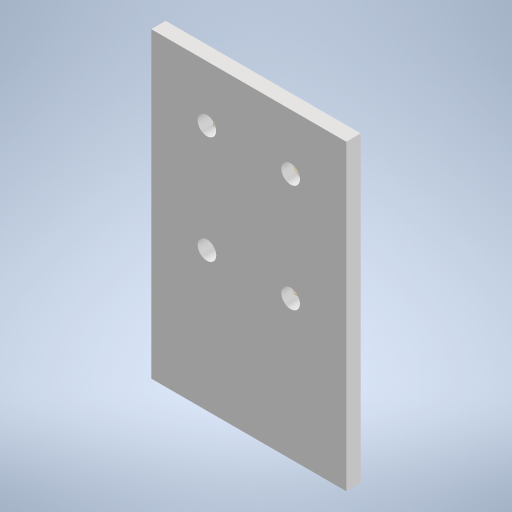
# Autodesk Inventor part: _Tooling_PCBPaste
Saved by Autodesk Inventor 2023.2 (Build 272271030, 271C)
## iProperties
Created: 2023-03-08
Part Number: _Tooling_PCBPaste
Material: Generic
Document SubType Name: Modeling
Designer: atrus
Density: 1 g/cm^3
Appearance: Default
Author: atrus
Autodesk Inventor part; units mm, degrees
ref_plane "YZ Plane" through (0, 0, 0) normal (1, 0, 0) x (0, 1, 0)
ref_plane "XZ Plane" through (0, 0, 0) normal (0, 1, 0) x (-1, 0, 0)
ref_plane "XY Plane" through (0, 0, 0) normal (0, 0, 1) x (1, 0, 0)
ref_plane "Work Plane1" through (0, 0, 0) normal (0, 0, 1) x (1, 0, 0)
sketch "Sketch1" plane through (0, 0, 0) normal (0, 0, 1) x (1, 0, 0)
  circle A0 centre (15.9836, 21.7327) radius 1.632 construction
  circle A1 centre (-16.0164, 21.7327) radius 1.632 construction
  circle A2 centre (15.9836, -10.6173) radius 1.632 construction
  circle A3 centre (-16.0164, -10.6173) radius 1.632 construction
  line L0 (19, -24.5) -> (19, 24.5) construction
  line L1 (19, 24.5) -> (-19, 24.5) construction
  line L2 (-19, 24.5) -> (-19, -24.5) construction
  line L3 (-19, -24.5) -> (19, -24.5) construction
  line L4 (-19.1, 24.6) -> (19.1, 24.6)
  line L5 (19.1, 24.6) -> (19.1, -24.6)
  line L6 (19.1, -24.6) -> (-19.1, -24.6)
  line L7 (-19.1, -24.6) -> (-19.1, 24.6)
  circle A4 centre (-16.0164, 21.7327) radius 1.5319
  circle A5 centre (15.9836, 21.7327) radius 1.5319
  circle A6 centre (-16.0164, -10.6173) radius 1.5319
  circle A7 centre (15.9836, -10.6173) radius 1.5319
  line L8 (-44.5, 50) -> (44.5, 50)
  line L9 (44.5, 50) -> (44.5, -88.1)
  line L10 (44.5, -88.1) -> (-44.5, -88.1)
  line L11 (-44.5, -88.1) -> (-44.5, 50)
  point P0 (0, 0)
  dimension "d0" = 0.1
  dimension "d1" = 0.1
  dimension "d2" = 0.1
  dimension "d3" = 0.1
  dimension "d4" = 0.1
  dimension "d5" = 63.5
  dimension "d6" = 25.4
  dimension "d7" = 25.4
  dimension "d8" = 25.4
  constraints: 16 end point, 4 centre point, 2 parallel, 1 horizontal, 1 perpendicular, 3 other
  measures "d0" distance between parallel lines of L1 L4
  measures "d1" radial gap between concentric circles of A1 A4
  measures "d2" radial gap between concentric circles of A0 A5
  measures "d3" radial gap between concentric circles of A3 A6
  measures "d4" radial gap between concentric circles of A2 A7
  measures "d5" distance between parallel lines of L10 L6
  measures "d6" distance between parallel lines of L8 L4
  measures "d7" distance between parallel lines of L9 L5
  measures "d8" distance between parallel lines of L11 L7
extrude "Extrusion1" add sketch "Sketch1" against normal blind 1.6
sketch "Sketch2" plane through (0, 0, 0) normal (0, 0, 1) x (1, 0, 0)
  line L0 (-44.5, 50) -> (44.5, 50) projected
  line L1 (44.5, 50) -> (44.5, -88.1) projected
  line L2 (-44.5, 50) -> (44.5, 50)
  line L3 (44.5, 50) -> (44.5, -88.1)
  line L4 (44.5, -88.1) -> (-44.5, -88.1)
  line L5 (-44.5, -88.1) -> (-44.5, 50)
  point P0 (0, 0)
  constraints: 8 end point, 2 parallel, 1 horizontal, 1 perpendicular
extrude "Extrusion2" add sketch "Sketch2" along normal blind 5
sketch "Sketch3" plane through (0, 0, -1.6) normal (0, 0, -1) x (-1, 0, 0)
  line L0 (-19.1, 24.6) -> (-19.1, -24.6) projected
  circle A0 centre (-15.9836, 21.7327) radius 1.5319 projected
  circle A1 centre (-19.1, 24.6) radius 4.2348
  line L1 (-19.1, 24.6) -> (19.1, 24.6) projected
  circle A2 centre (16.0164, 21.7327) radius 1.5319 projected
  circle A3 centre (19.1, 24.6) radius 4.2107
  circle A4 centre (19.1, -24.6) radius 4.2348
  circle A5 centre (-19.1, -24.6) radius 4.2348
  point P0 (0, 0)
  constraints: 2 centre point, 1 coincident, 8 other
extrude "Extrusion3" cut sketch "Sketch3" against normal through all contours L1 A1 A0 L0 | L0 A1 L1 | A0 A1 | A2 A3 | A2 A3 | A4 | A5 picked at (-16.3746, 22.0925) picked at (16.4181, 22.0806) picked at (20.3065, 26.0638)
sketch "Sketch4" plane through (0, 0, -1.6) normal (0, 0, -1) x (-1, 0, 0)
  line L0 (37.9315, -14.1978) -> (37.9315, 20.0606) construction
  line L1 (37.9315, 20.0606) -> (45.2777, 20.0606) construction
  line L2 (45.2777, 20.0606) -> (45.2777, -14.1978) construction
  line L3 (45.2777, -14.1978) -> (37.9315, -14.1978) construction
  line L4 (41.1606, -12.3998) -> (39.2658, -13.2505)
  line L5 (39.2658, -13.2505) -> (38.859, -13.4268)
  line L6 (38.859, -13.4268) -> (40.1734, -13.4268)
  line L7 (40.1734, -13.4268) -> (41.1606, -13.4268)
  line L8 (41.1606, -13.4268) -> (41.1606, -13.9702)
  line L9 (41.1606, -13.9702) -> (37.9856, -13.9702)
  line L10 (37.9856, -13.9702) -> (37.9856, -13.2362)
  line L11 (37.9856, -13.2362) -> (39.8917, -12.3685)
  line L12 (39.8917, -12.3685) -> (40.2644, -12.2149)
  line L13 (40.2644, -12.2149) -> (38.8618, -12.2149)
  line L14 (38.8618, -12.2149) -> (37.9856, -12.2149)
  line L15 (37.9856, -12.2149) -> (37.9856, -11.6715)
  line L16 (37.9856, -11.6715) -> (41.1606, -11.6715)
  line L17 (41.1606, -11.6715) -> (41.1606, -12.3998)
  line L18 (41.1606, -9.5747) -> (40.8391, -9.589)
  spline S0 degree 2 poles (40.8391, -9.589) (40.9216, -9.6686) (41.0582, -9.8365) (41.1606, -10.0413) (41.2175, -10.2831) (41.2175, -10.4254) knots 0 0 0 1 2 3 4 4 4
  spline S1 degree 2 poles (41.2175, -10.4254) (41.2175, -10.616) (41.1065, -10.9033) (40.9074, -11.0968) (40.6229, -11.1964) (40.455, -11.1964) knots 0 0 0 1 2 3 4 4 4
  spline S2 degree 2 poles (40.455, -11.1964) (40.2786, -11.1964) (39.9827, -11.0484) (39.7694, -10.744) (39.647, -10.2888) (39.647, -9.9844) knots 0 0 0 1 2 3 4 4 4
  line L19 (39.647, -9.9844) -> (39.647, -9.6601)
  line L20 (39.647, -9.6601) -> (39.4991, -9.6601)
  spline S3 degree 2 poles (39.4991, -9.6601) (39.4052, -9.6601) (39.2516, -9.7141) (39.1435, -9.8336) (39.0866, -10.0214) (39.0866, -10.1608) knots 0 0 0 1 2 3 4 4 4
  spline S4 degree 2 poles (39.0866, -10.1608) (39.0866, -10.3799) (39.1862, -10.8038) (39.2772, -11.0029) knots 0 0 0 1 2 2 2
  line L21 (39.2772, -11.0029) -> (38.8021, -11.0029)
  spline S5 degree 2 poles (38.8021, -11.0029) (38.731, -10.8265) (38.6399, -10.3628) (38.6399, -10.1124) knots 0 0 0 1 2 2 2
  spline S6 degree 2 poles (38.6399, -10.1124) (38.6399, -9.8365) (38.7452, -9.4439) (38.9529, -9.1907) (39.2658, -9.0683) (39.4763, -9.0683) knots 0 0 0 1 2 3 4 4 4
  line L22 (39.4763, -9.0683) -> (41.1606, -9.0683)
  line L23 (41.1606, -9.0683) -> (41.1606, -9.5747)
  line L24 (40.0709, -9.6601) -> (40.0709, -10.0214)
  spline S7 degree 2 poles (40.0709, -10.0214) (40.0709, -10.1722) (40.1278, -10.3827) (40.2303, -10.5136) (40.364, -10.5733) (40.4408, -10.5733) knots 0 0 0 1 2 3 4 4 4
  spline S8 degree 2 poles (40.4408, -10.5733) (40.5916, -10.5733) (40.748, -10.3799) (40.748, -10.212) knots 0 0 0 1 2 2 2
  spline S9 degree 2 poles (40.748, -10.212) (40.748, -10.0868) (40.5688, -9.8194) (40.401, -9.6601) knots 0 0 0 1 2 2 2
  line L25 (40.401, -9.6601) -> (40.0709, -9.6601)
  line L26 (41.1606, -6.9118) -> (39.5532, -6.9118)
  spline S10 degree 2 poles (39.5532, -6.9118) (39.1463, -6.9118) (39.1463, -7.2134) knots 0 0 0 1 1 1
  spline S11 degree 2 poles (39.1463, -7.2134) (39.1463, -7.3642) (39.3881, -7.6401) (39.5987, -7.7938) knots 0 0 0 1 2 2 2
  line L27 (39.5987, -7.7938) -> (41.1606, -7.7938)
  line L28 (41.1606, -7.7938) -> (41.1606, -8.3855)
  line L29 (41.1606, -8.3855) -> (38.6911, -8.3855)
  line L30 (38.6911, -8.3855) -> (38.6911, -7.8734)
  line L31 (38.6911, -7.8734) -> (39.0553, -7.8592)
  spline S12 degree 2 poles (39.0553, -7.8592) (38.9614, -7.7852) (38.8078, -7.6202) (38.6968, -7.4325) (38.6399, -7.2134) (38.6399, -7.0768) knots 0 0 0 1 2 3 4 4 4
  spline S13 degree 2 poles (38.6399, -7.0768) (38.6399, -6.8862) (38.7651, -6.6046) (38.9898, -6.414) (39.3085, -6.3201) (39.5048, -6.3201) knots 0 0 0 1 2 3 4 4 4
  line L32 (39.5048, -6.3201) -> (41.1606, -6.3201)
  line L33 (41.1606, -6.3201) -> (41.1606, -6.9118)
  spline S14 degree 2 poles (39.9088, -3.4267) (40.199, -3.4267) (40.6826, -3.5917) (41.0269, -3.9018) (41.2175, -4.3542) (41.2175, -4.6444) knots 0 0 0 1 2 3 4 4 4
  spline S15 degree 2 poles (41.2175, -4.6444) (41.2175, -4.9203) (41.0582, -5.3528) (40.7395, -5.6543) (40.2616, -5.8137) (39.9429, -5.8137) knots 0 0 0 1 2 3 4 4 4
  spline S16 degree 2 poles (39.9429, -5.8137) (39.647, -5.8137) (39.1662, -5.6458) (38.8277, -5.3329) (38.6399, -4.8805) (38.6399, -4.596) knots 0 0 0 1 2 3 4 4 4
  spline S17 degree 2 poles (38.6399, -4.596) (38.6399, -4.3201) (38.8021, -3.8848) (39.1236, -3.586) (39.5958, -3.4267) (39.9088, -3.4267) knots 0 0 0 1 2 3 4 4 4
  spline S18 degree 2 poles (39.923, -4.0441) (39.5389, -4.0441) (39.152, -4.3343) (39.152, -4.6159) knots 0 0 0 1 2 2 2
  spline S19 degree 2 poles (39.152, -4.6159) (39.152, -4.7696) (39.2743, -4.9886) (39.4849, -5.1309) (39.7665, -5.1963) (39.9287, -5.1963) knots 0 0 0 1 2 3 4 4 4
  spline S20 degree 2 poles (39.9287, -5.1963) (40.3128, -5.1963) (40.7054, -4.8862) (40.7054, -4.6159) knots 0 0 0 1 2 2 2
  spline S21 degree 2 poles (40.7054, -4.6159) (40.7054, -4.468) (40.5859, -4.2489) (40.3754, -4.1124) (40.088, -4.0441) (39.923, -4.0441) knots 0 0 0 1 2 3 4 4 4
  line L34 (41.1606, -2.9374) -> (37.9856, -2.9374)
  line L35 (37.9856, -2.9374) -> (37.9856, -1.9132)
  spline S22 degree 2 poles (37.9856, -1.9132) (37.9856, -1.3698) (38.364, -0.8293) (38.748, -0.8293) knots 0 0 0 1 2 2 2
  spline S23 degree 2 poles (38.748, -0.8293) (38.8647, -0.8293) (39.0923, -0.8862) (39.28, -1.0028) (39.4251, -1.1763) (39.4678, -1.2958) knots 0 0 0 1 2 3 4 4 4
  spline S24 degree 2 poles (39.4678, -1.2958) (39.4877, -1.1763) (39.6015, -0.9601) (39.7836, -0.798) (40.0311, -0.7041) (40.1847, -0.7041) knots 0 0 0 1 2 3 4 4 4
  spline S25 degree 2 poles (40.1847, -0.7041) (40.6712, -0.7041) (41.1606, -1.3556) (41.1606, -1.9701) knots 0 0 0 1 2 2 2
  line L36 (41.1606, -1.9701) -> (41.1606, -2.9374)
  spline S26 degree 2 poles (40.6712, -1.9274) (40.6712, -1.7852) (40.5973, -1.569) (40.4692, -1.421) (40.2957, -1.347) (40.1961, -1.347) knots 0 0 0 1 2 3 4 4 4
  spline S27 degree 2 poles (40.1961, -1.347) (39.9884, -1.347) (39.7551, -1.6543) (39.7551, -1.9729) knots 0 0 0 1 2 2 2
  line L37 (39.7551, -1.9729) -> (39.7551, -2.3456)
  line L38 (39.7551, -2.3456) -> (40.6712, -2.3456)
  line L39 (40.6712, -2.3456) -> (40.6712, -1.9274)
  spline S28 degree 2 poles (38.8533, -1.4523) (38.7622, -1.4523) (38.6172, -1.5092) (38.5176, -1.6401) (38.4607, -1.8421) (38.4607, -1.9843) knots 0 0 0 1 2 3 4 4 4
  line L40 (38.4607, -1.9843) -> (38.4607, -2.3456)
  line L41 (38.4607, -2.3456) -> (39.2971, -2.3456)
  line L42 (39.2971, -2.3456) -> (39.2971, -1.9843)
  spline S29 degree 2 poles (39.2971, -1.9843) (39.2971, -1.8392) (39.226, -1.6372) (39.1036, -1.5092) (38.9443, -1.4523) (38.8533, -1.4523) knots 0 0 0 1 2 3 4 4 4
  spline S30 degree 2 poles (39.9088, 2.047) (40.199, 2.047) (40.6826, 1.882) (41.0269, 1.5719) (41.2175, 1.1196) (41.2175, 0.8294) knots 0 0 0 1 2 3 4 4 4
  spline S31 degree 2 poles (41.2175, 0.8294) (41.2175, 0.5534) (41.0582, 0.121) (40.7395, -0.1806) (40.2616, -0.3399) (39.9429, -0.3399) knots 0 0 0 1 2 3 4 4 4
  spline S32 degree 2 poles (39.9429, -0.3399) (39.647, -0.3399) (39.1662, -0.1721) (38.8277, 0.1409) (38.6399, 0.5932) (38.6399, 0.8777) knots 0 0 0 1 2 3 4 4 4
  spline S33 degree 2 poles (38.6399, 0.8777) (38.6399, 1.1537) (38.8021, 1.589) (39.1236, 1.8877) (39.5958, 2.047) (39.9088, 2.047) knots 0 0 0 1 2 3 4 4 4
  spline S34 degree 2 poles (39.923, 1.4297) (39.5389, 1.4297) (39.152, 1.1395) (39.152, 0.8578) knots 0 0 0 1 2 2 2
  spline S35 degree 2 poles (39.152, 0.8578) (39.152, 0.7042) (39.2743, 0.4851) (39.4849, 0.3429) (39.7665, 0.2774) (39.9287, 0.2774) knots 0 0 0 1 2 3 4 4 4
  spline S36 degree 2 poles (39.9287, 0.2774) (40.3128, 0.2774) (40.7054, 0.5875) (40.7054, 0.8578) knots 0 0 0 1 2 2 2
  spline S37 degree 2 poles (40.7054, 0.8578) (40.7054, 1.0058) (40.5859, 1.2248) (40.3754, 1.3614) (40.088, 1.4297) (39.923, 1.4297) knots 0 0 0 1 2 3 4 4 4
  line L43 (41.1606, 4.1495) -> (40.327, 3.589)
  line L44 (40.327, 3.589) -> (41.1606, 3.02)
  line L45 (41.1606, 3.02) -> (41.1606, 2.3059)
  line L46 (41.1606, 2.3059) -> (39.9173, 3.2277)
  line L47 (39.9173, 3.2277) -> (38.6911, 2.3543)
  line L48 (38.6911, 2.3543) -> (38.6911, 3.0769)
  line L49 (38.6911, 3.0769) -> (39.5048, 3.6288)
  line L50 (39.5048, 3.6288) -> (38.6911, 4.1751)
  line L51 (38.6911, 4.1751) -> (38.6911, 4.8408)
  line L52 (38.6911, 4.8408) -> (39.9116, 3.9901)
  line L53 (39.9116, 3.9901) -> (41.1606, 4.8863)
  line L54 (41.1606, 4.8863) -> (41.1606, 4.1495)
  line L55 (41.1606, 9.4155) -> (41.1606, 8.7327)
  line L56 (41.1606, 8.7327) -> (38.6911, 7.7569)
  line L57 (38.6911, 7.7569) -> (38.6911, 8.4169)
  line L58 (38.6911, 8.4169) -> (40.0937, 8.929)
  line L59 (40.0937, 8.929) -> (40.5461, 9.0827)
  line L60 (40.5461, 9.0827) -> (40.1108, 9.2334)
  line L61 (40.1108, 9.2334) -> (38.6911, 9.7512)
  line L62 (38.6911, 9.7512) -> (38.6911, 10.3885)
  line L63 (38.6911, 10.3885) -> (41.1606, 9.4155)
  spline S38 degree 2 poles (40.1904, 12.912) (40.4266, 12.912) (40.8021, 12.7385) (41.0667, 12.3743) (41.2089, 11.8252) (41.2089, 11.4554) knots 0 0 0 1 2 3 4 4 4
  spline S39 degree 2 poles (41.2089, 11.4554) (41.2089, 11.3729) (41.2004, 11.1908) (41.189, 11.0116) (41.1719, 10.8409) (41.1606, 10.7726) knots 0 0 0 1 2 3 4 4 4
  line L64 (41.1606, 10.7726) -> (40.6456, 10.7726)
  spline S40 degree 2 poles (40.6456, 10.7726) (40.6741, 10.9262) (40.7111, 11.3074) (40.7111, 11.5123) knots 0 0 0 1 2 2 2
  spline S41 degree 2 poles (40.7111, 11.5123) (40.7111, 11.7143) (40.6428, 12.0073) (40.5148, 12.1951) (40.3241, 12.2861) (40.2047, 12.2861) knots 0 0 0 1 2 3 4 4 4
  spline S42 degree 2 poles (40.2047, 12.2861) (40.1022, 12.2861) (39.9315, 12.1951) (39.812, 12.0045) (39.7466, 11.7114) (39.7466, 11.5094) knots 0 0 0 1 2 3 4 4 4
  line L65 (39.7466, 11.5094) -> (39.7466, 11.1567)
  line L66 (39.7466, 11.1567) -> (39.2943, 11.1567)
  line L67 (39.2943, 11.1567) -> (39.2943, 11.4781)
  spline S43 degree 2 poles (39.2943, 11.4781) (39.2943, 11.6687) (39.2203, 11.9191) (39.0923, 12.067) (38.9187, 12.1296) (38.8248, 12.1296) knots 0 0 0 1 2 3 4 4 4
  spline S44 degree 2 poles (38.8248, 12.1296) (38.6314, 12.1296) (38.4294, 11.8764) (38.4294, 11.6118) knots 0 0 0 1 2 2 2
  spline S45 degree 2 poles (38.4294, 11.6118) (38.4294, 11.4241) (38.5034, 11.0542) (38.5631, 10.8579) knots 0 0 0 1 2 2 2
  line L68 (38.5631, 10.8579) -> (38.0652, 10.8579)
  spline S46 degree 2 poles (38.0652, 10.8579) (38.0282, 10.966) (37.9799, 11.1652) (37.9457, 11.3643) (37.9315, 11.5692) (37.9315, 11.6773) knots 0 0 0 1 2 3 4 4 4
  spline S47 degree 2 poles (37.9315, 11.6773) (37.9315, 11.939) (38.0425, 12.3373) (38.2502, 12.6047) (38.546, 12.7413) (38.7281, 12.7413) knots 0 0 0 1 2 3 4 4 4
  spline S48 degree 2 poles (38.7281, 12.7413) (39.0183, 12.7413) (39.3739, 12.4767) (39.4707, 12.2377) knots 0 0 0 1 2 2 2
  spline S49 degree 2 poles (39.4707, 12.2377) (39.4934, 12.3914) (39.6129, 12.6389) (39.8007, 12.8181) (40.0425, 12.912) (40.1904, 12.912) knots 0 0 0 1 2 3 4 4 4
  line L69 (41.1606, 13.5407) -> (40.6342, 13.5407)
  line L70 (40.6342, 13.5407) -> (40.6342, 14.3487)
  line L71 (40.6342, 14.3487) -> (38.5916, 14.3487)
  line L72 (38.5916, 14.3487) -> (38.9813, 13.6432)
  line L73 (38.9813, 13.6432) -> (38.4977, 13.4497)
  line L74 (38.4977, 13.4497) -> (37.9657, 14.4568)
  line L75 (37.9657, 14.4568) -> (37.9657, 14.9575)
  line L76 (37.9657, 14.9575) -> (40.6342, 14.9575)
  line L77 (40.6342, 14.9575) -> (40.6342, 15.6546)
  line L78 (40.6342, 15.6546) -> (41.1606, 15.6546)
  line L79 (41.1606, 15.6546) -> (41.1606, 13.5407)
  point P0 (0, 0)
  constraints: 2 other
emboss "Emboss1" sketch "Sketch4" operation cut depth 0.2 direction (0, 0, 1)
body "Solid1"
